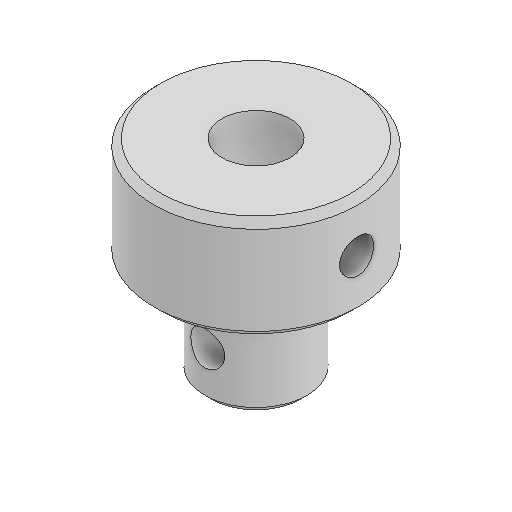
# Autodesk Inventor part: Acople_EJE
Saved by Autodesk Inventor 2025 (Build 290162000, 162)
## iProperties
Created: 2026-02-06
Part Number: Acople_EJE
Material: Genérico
Document SubType Name: Modeling
Designer: HP
Density: 1 g/cm^3
Appearance: Valor por defecto
Author: HP
Autodesk Inventor part; units mm, degrees
ref_plane "XZ Plane" through (0, 0, 0) normal (0, 1, 0) x (-1, 0, 0)
sketch "Boceto1" plane through (0, 0, 0) normal (0, 1, 0) x (-1, 0, 0)
  circle A0 centre (0, 0) radius 15
  dimension "d0" = 30
  constraints: 1 centre point, 1 coincident
  measures "d0" diameter of A0
extrude "Extrusión1" add sketch "Boceto1" along normal blind 10
sketch "Boceto2" plane through (0, 10, 0) normal (0, 1, 0) x (1, 0, 0)
  circle A0 centre (0, 0) radius 5
  dimension "d3" = 10
  constraints: 1 centre point, 1 coincident
  measures "d3" diameter of A0
extrude "Extrusión2" cut sketch "Boceto2" against normal blind 5
sketch "Boceto3" plane through (0, 0, 0) normal (0, -1, 0) x (1, 0, 0)
  circle A0 centre (0, 0) radius 7.5
  dimension "d6" = 15
  constraints: 1 centre point, 1 coincident
  measures "d6" diameter of A0
extrude "Extrusión3" add sketch "Boceto3" along normal blind 10
sketch "Boceto4" plane through (0, -10, 0) normal (0, -1, 0) x (1, 0, 0)
  circle A0 centre (0, 0) radius 2.975
  dimension "d9" = 5.95
  constraints: 1 centre point, 1 coincident
  measures "d9" diameter of A0
extrude "Extrusión4" cut sketch "Boceto4" against normal blind 5
sketch "Boceto5" plane through (0, 10, 0) normal (0, 1, 0) x (1, 0, 0)
  circle A0 centre (0, 0) radius 5 projected
  circle A1 centre (0, 0) radius 15 projected
extrude "Extrusión5" add sketch "Boceto5" along normal blind 5
sketch "Boceto6" plane through (0, -10, 0) normal (0, -1, 0) x (1, 0, 0)
  circle A0 centre (0, 0) radius 2.975 projected
  circle A1 centre (0, 0) radius 7.5 projected
extrude "Extrusión6" add sketch "Boceto6" along normal blind 5
chamfer "Chaflán1" distance 1 angle 45 1 edges at (-7.5, -15, 0)
chamfer "Chaflán2" distance 1 angle 45 1 edges at (15, 0, 0)
chamfer "Chaflán3" distance 1 angle 45 1 edges at (-15, 15, 0)
fillet "Empalme1" radius 2 1 edges at (-7.5, 0, 0)
ref_plane "Plano de trabajo1" through (15, 0, 0) normal (1, 0, 0) x (0, 1, 0)
sketch "Boceto7" plane through (15, 0, 0) normal (1, 0, 0) x (0, 1, 0)
  line L0 (1, 15) -> (1, -15) projected
  line L1 (14, -15) -> (14, 15) projected
  line L2 (1, -15) -> (14, -15) projected
  line L3 (1, 15) -> (14, 15) projected
  line L4 (7.5, 15) -> (7.5, -15) construction
  circle A0 centre (7.5, 0) radius 2.5
  point P0 (0, 0)
  dimension "d27" = 5
  constraints: 3 midpoint, 2 end point, 1 centre point
  measures "d27" diameter of A0
extrude "Extrusión7" cut sketch "Boceto7" against normal blind 11 contours A0
ref_plane "Plano de trabajo2" through (0, 0, 7.5) normal (0, 0, 1) x (1, 0, 0)
sketch "Boceto8" plane through (0, 0, 7.5) normal (0, 0, 1) x (1, 0, 0)
  line L0 (-7.5, -14) -> (7.5, -14) projected
  line L1 (7.5, -2) -> (-7.5, -2) projected
  line L2 (7.5, -2) -> (7.5, -14) projected
  line L3 (-7.5, -2) -> (-7.5, -14) projected
  line L4 (7.5, -8) -> (-7.5, -8) construction
  circle A0 centre (0, -8) radius 2.5
  point P0 (0, 0)
  dimension "d31" = 5
  constraints: 3 midpoint, 2 end point, 1 centre point
  measures "d31" diameter of A0
extrude "Extrusión8" cut sketch "Boceto8" against normal blind 6 contours A0
